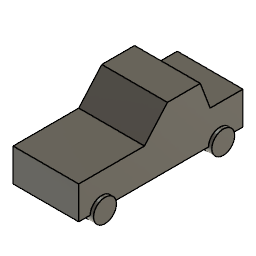
car (Autodesk Fusion 360 design; units mm, degrees)
Autodesk Fusion 360 part; units mm, degrees
note: some values were not read from the file. Set by a fixed rule: which sketch regions a step uses.
sketch "スケッチ1" plane through (0, 0, 0) normal (1, 0, 0) x (0, 1, 0)
  line L0 (0, 0) -> (0, 10)
  line L1 (0, 10) -> (20, 10)
  line L2 (20, 10) -> (20, 18)
  line L3 (20, 18) -> (40, 18)
  line L4 (40, 18) -> (40, 10)
  line L5 (40, 10) -> (50, 10)
  line L6 (50, 10) -> (50, 0)
  line L7 (50, 0) -> (0, 0)
  dimension "d1" = 10
  dimension "d2" = 10
  dimension "d3" = 20
  dimension "d4" = 8
  dimension "d5" = 10
  dimension "d6" = 20
  constraint coincident L0.start L7.end
  constraint vertical L0
  constraint perpendicular L0 L1
  constraint perpendicular L1 L2
  constraint perpendicular L2 L3
  constraint perpendicular L3 L4
  constraint perpendicular L2 L5
  constraint perpendicular L5 L6
  constraint horizontal L7
  measures "d1" distance of L0.start L0.end
  measures "d2" distance of L5.end L6.end
  measures "d3" distance of L2.end L3.end
  measures "d4" distance of L1.end L2.end
  measures "d5" distance of L4.end L5.end
  measures "d6" distance of L0.end L1.end
extrude "押し出し1" add sketch "スケッチ1" along normal blind 20
sketch "スケッチ2" plane through (20, 0, 0) normal (1, 0, 0) x (0, 1, 0)
  line L0 (50, 0) -> (50, 10)
  line L1 (50, 10) -> (40, 10)
  line L2 (40, 10) -> (40, 18)
  line L3 (40, 18) -> (20, 18)
  line L4 (20, 18) -> (20, 10)
  line L5 (20, 10) -> (0, 10)
  line L6 (0, 10) -> (0, 0)
  line L7 (0, 0) -> (50, 0)
  circle A0 centre (7, 0) radius 3.5
  circle A1 centre (43, 0) radius 3.5
  dimension "d9" = 7
  dimension "d10" = 7
  dimension "d11" = 7
  dimension "d12" = 7
  constraint coincident L7 A0.centre
  constraint coincident L7 A1.centre
  measures "d9" diameter of A0
  measures "d10" diameter of A1
  measures "d11" distance of L6.end A0.centre
  measures "d12" distance of L0.start A1.centre
extrude "押し出し2" add sketch "スケッチ2" along normal blind 1 and the other way blind 2 contours L7 A1 | L7 A1 | L7 A0 | L7 A0
ref_plane "作業平面1" through (10, 25, 9) normal (1, 0, 0) x (0, 0, -1)
mirror "ミラー1" about plane through (10, 25, 9) normal (1, 0, 0) of "押し出し2"
sketch "スケッチ3" plane through (20, 0, 0) normal (1, 0, 0) x (0, 1, 0)
  arc A0 (46.5, 0) -> (39.5, 0) centre (43, 0) ccw
  line L0 (46.5, 0) -> (50, 0)
  line L1 (50, 0) -> (50, 10)
  line L2 (50, 10) -> (40, 10)
  line L3 (40, 10) -> (40, 18)
  line L4 (40, 18) -> (20, 18)
  line L5 (20, 18) -> (20, 10)
  line L6 (20, 10) -> (0, 10)
  line L7 (0, 10) -> (0, 0)
  line L8 (0, 0) -> (3.5, 0)
  arc A1 (10.5, 0) -> (3.5, 0) centre (7, 0) ccw
  line L9 (10.5, 0) -> (39.5, 0)
  line L10 (20, 10) -> (27, 18)
  line L11 (40, 10) -> (37, 18)
  dimension "d19" = 7
  dimension "d20" = 3
  constraint coincident L5.end L6.start
  constraint coincident L4 L10.end
  constraint coincident L2.end L3.start
  constraint coincident L4 L11.end
  measures "d19" distance of L4.end L10.end
  measures "d20" distance of L3.end L11.end
extrude "押し出し3" cut sketch "スケッチ3" against normal blind 20 contours L3 L4 L11 | L4 L5 L10
